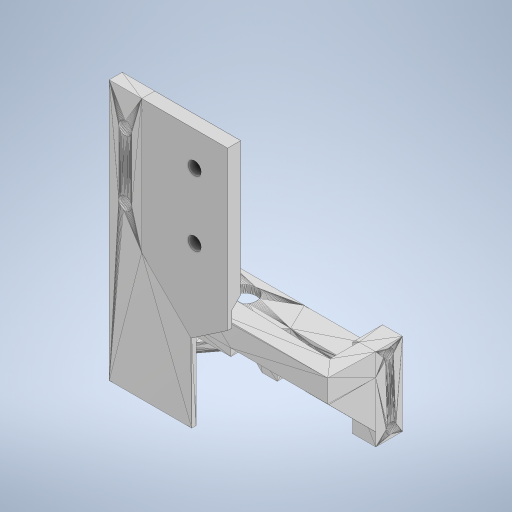
# Autodesk Inventor part: крепежная основа_спасена
Saved by Autodesk Inventor 2024.2 (Build 282272000, 272)
## iProperties
Created: 2026-03-03
Part Number: крепежная основа_спасена
Material: Типовые
Document SubType Name: Modeling
Designer: Service
Density: 1 g/cm^3
Appearance: По умолчанию
Author: Service
Autodesk Inventor part; units mm, degrees
ref_plane "YZ Plane" through (0, 0, 0) normal (1, 0, 0) x (0, 1, 0)
ref_plane "XZ Plane" through (0, 0, 0) normal (0, 1, 0) x (-1, 0, 0)
ref_plane "XY Plane" through (0, 0, 0) normal (0, 0, 1) x (1, 0, 0)
sketch "Эскиз1" plane through (40.6168, 2.0533, -8.0979) normal (1, 0, 0) x (0, 1, 0)
  line L0 (0.0252, 10.8303) -> (-10.8412, -0.0136)
  line L1 (-10.8412, -0.0136) -> (0.0252, -0.0136)
  line L2 (0.0252, -0.0136) -> (0.0252, 10.8303)
  point P0 (-2.0533, 8.0979)
  constraints: 6 end point, 1 horizontal, 1 perpendicular
extrude "Выдавливание1" add sketch "Эскиз1" against normal blind 5.358
sketch "Эскиз2" plane through (4.4799, 48.5533, 9.6685) normal (0, 0, 1) x (1, 0, 0)
  line L0 (11.25, -42) -> (0, -30.75) projected
  line L1 (0, -30.75) -> (0, 0) projected
  line L2 (0, 0) -> (-7.4799, 0) projected
  line L3 (11.5201, -60) -> (11.5201, -42) projected
  line L4 (11.25, -42) -> (11.5201, -42) projected
  line L5 (0, 0) -> (19.7943, 0)
  line L6 (19.7943, 0) -> (19.7943, -36.375)
  line L7 (19.7943, -36.375) -> (5.625, -36.375)
  circle A0 centre (-3.7947, -7.8002) radius 1.5003 projected
  circle A1 centre (-3.7949, -22.8) radius 1.5 projected
  circle A2 centre (12.2053, -7.8) radius 1.5
  circle A3 centre (12.2051, -22.8) radius 1.5
  line L8 (11.5201, -42) -> (19.7943, -36.375)
  line L9 (-0.1192, -30.8692) -> (0, -30.75)
  line L10 (19.7943, -30.75) -> (0, -30.75)
  line L11 (19.7943, -30.75) -> (11.5201, -42)
  point P0 (-4.4799, -48.5533)
  point P1 (15.6572, -36.375)
  dimension "d2" = 3
  dimension "d3" = 3
  dimension "d4" = 16
  dimension "d5" = 16
  dimension "d6" = 13.575
  dimension "d7" = 13.575
  dimension "d8" = 15
  constraints: 14 end point, 2 centre point, 2 horizontal, 1 midpoint, 1 perpendicular, 1 point on line
  measures "d2" diameter of A3
  measures "d3" diameter of A2
  measures "d4" distance of A0.centre A2.centre
  measures "d5" distance of A1.centre A3.centre
  measures "d6" distance from line of L7 A1.centre
  measures "d7" distance from line of L7 A3.centre
  measures "d8" distance of A2.centre A3.centre
extrude "Выдавливание2" add sketch "Эскиз2" against normal blind 3 contours L1 L5 L6 L10
extrude "Выдавливание3" add sketch "Эскиз2" against normal blind 1 contours L0 L7 L11 L4 | L0 L10 L11 L7 | L11 L7 L8 | L11 L6 L7
chamfer "Фаска1" distance 2 angle 45 1 edges at (14.377, 17.8033, 8.6685)
